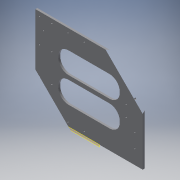
# Autodesk Inventor part: BasePlate
Saved by Autodesk Inventor 2016 (Build 200138000, 138)
## iProperties
Created: 2016-04-23
Part Number: BasePlate
Material: Generic
Document SubType Name: Modeling
Designer: Scott
Density: 1 g/cm^3
Appearance: Default
Author: Scott
Autodesk Inventor part; units mm, degrees
ref_plane "YZ Plane" through (0, 0, 0) normal (1, 0, 0) x (0, 1, 0)
ref_plane "XZ Plane" through (0, 0, 0) normal (0, 1, 0) x (-1, 0, 0)
ref_plane "XY Plane" through (0, 0, 0) normal (0, 0, 1) x (1, 0, 0)
ref_plane "Work Plane1" through (0, 0, 0) normal (0, 0, 1) x (1, 0, 0)
sketch "Sketch1" plane through (0, 0, 0) normal (0, 0, 1) x (1, 0, 0)
  line L0 (0, 273.904) -> (158.3386, 273.904)
  line L1 (133.9788, 273.904) -> (133.9788, 6.096)
  line L2 (-34.2962, 6.096) -> (302.2538, 6.096)
  line L3 (302.2538, 6.096) -> (302.2538, 273.904)
  line L4 (302.2538, 273.904) -> (-34.2962, 273.904)
  line L5 (-34.2962, 273.904) -> (-34.2962, 6.096)
  line L6 (-34.2962, 6.096) -> (302.2538, 273.904) construction
  line L7 (302.2538, 6.096) -> (-34.2962, 273.904) construction
  point P0 (0, 0)
  point P1 (0, 6.096)
  point P2 (133.9788, 140)
  dimension "d0" = 336.55
  constraints: 16 end point, 3 midpoint, 2 horizontal, 2 parallel, 1 perpendicular, 1 point on line, 1 vertical, 2 other
  measures "d0" distance of L4.end L3.end
extrude "Extrusion1" add sketch "Sketch1" against normal blind 6.096
sketch "Sketch2" plane through (0, 0, -6.096) normal (0, 0, -1) x (-1, 0, 0)
  line L0 (-302.2538, 6.096) -> (34.2962, 6.096) projected
  line L1 (34.2962, 6.096) -> (34.2962, 273.904) projected
  line L2 (34.2962, 273.904) -> (-302.2538, 273.904) projected
  line L3 (-302.2538, 273.904) -> (-302.2538, 6.096) projected
  line L4 (34.2962, 6.096) -> (-16.5038, 6.096)
  line L5 (-302.2538, 6.096) -> (34.2962, 6.096) projected
  line L6 (-16.5038, 6.096) -> (-67.3038, 6.096)
  line L7 (-67.3038, 6.096) -> (-118.1038, 6.096)
  line L8 (-16.5038, 6.096) -> (-16.5038, 18.796)
  circle A0 centre (-16.5038, 18.796) radius 2.2225
  circle A1 centre (-118.1038, 18.796) radius 2.2225
  circle A2 centre (-67.3038, 18.796) radius 2.2225
  line L9 (-16.5038, 18.796) -> (21.5962, 18.796)
  circle A3 centre (21.5962, 18.796) radius 2.2225
  line L10 (34.2962, 6.096) -> (34.2962, 273.904) projected
  line L11 (34.2962, 140) -> (8.8962, 140)
  line L12 (34.2962, 273.904) -> (-16.5038, 273.904)
  line L13 (-16.5038, 273.904) -> (-67.3038, 273.904)
  line L14 (-67.3038, 273.904) -> (-118.1038, 273.904)
  line L15 (-16.5038, 273.904) -> (-16.5038, 261.204)
  circle A4 centre (-16.5038, 261.204) radius 2.2225
  circle A5 centre (-118.1038, 261.204) radius 2.2225
  circle A6 centre (-67.3038, 261.204) radius 2.2225
  line L16 (-16.5038, 261.204) -> (21.5962, 261.204)
  circle A7 centre (21.5962, 261.204) radius 2.2225
  point P0 (0, 0)
  point P1 (0, 280)
  dimension "d3" = 50.8
  dimension "d4" = 50.8
  dimension "d5" = 50.8
  dimension "d6" = 12.7
  dimension "d7" = 4.445
  dimension "d8" = 4.445
  dimension "d9" = 4.445
  dimension "d10" = 38.1
  dimension "d11" = 4.445
  constraints: 22 end point, 10 symmetric about line, 8 centre point, 4 coincident, 3 point on line, 2 horizontal, 1 midpoint, 1 vertical, 4 other
  measures "d3" distance of L0.end L4.end
  measures "d4" distance of L4.end L6.end
  measures "d5" distance of L6.end L7.end
  measures "d6" distance of L4.end L8.end
  measures "d7" diameter of A0
  measures "d8" diameter of A1
  measures "d9" diameter of A2
  measures "d10" distance of L9.start L9.end
  measures "d11" diameter of A3
extrude "Extrusion2" cut sketch "Sketch2" against normal blind 10.8585 contours A0 L9 L8 | L8 L9 A0 | A1 | A2 | A3 | A4 L16 L15 | L15 L16 A4 | A5 | A6 | A7
sketch "Sketch3" plane through (0, 0, -6.096) normal (0, 0, -1) x (-1, 0, 0)
  circle A0 centre (-67.3038, 261.204) radius 2.2225 projected
  circle A1 centre (21.5962, 261.204) radius 2.2225 projected
  circle A2 centre (-67.3038, 18.796) radius 2.2225 projected
  circle A3 centre (-16.5038, 18.796) radius 2.2225 projected
  circle A4 centre (-118.1038, 18.796) radius 2.2225 projected
  circle A5 centre (21.5962, 18.796) radius 2.2225 projected
  circle A6 centre (-16.5038, 261.204) radius 2.2225 projected
  circle A7 centre (-118.1038, 261.204) radius 2.2225 projected
  line L0 (-302.2538, 6.096) -> (34.2962, 6.096) projected
  line L1 (34.2962, 6.096) -> (34.2962, 273.904) projected
  line L2 (34.2962, 273.904) -> (-302.2538, 273.904) projected
  line L3 (-302.2538, 273.904) -> (-302.2538, 6.096) projected
  circle A8 centre (8.8962, 228.9) radius 2.2225
  circle A9 centre (21.5962, 184.45) radius 2.2225
  circle A10 centre (-16.5038, 184.45) radius 2.2225
  circle A11 centre (-16.5038, 95.55) radius 2.2225
  circle A12 centre (8.8962, 51.1) radius 2.2225
  circle A13 centre (21.5962, 95.55) radius 2.2225
  point P0 (0, 0)
  dimension "d20" = 4.445
  dimension "d21" = 4.445
  dimension "d22" = 4.445
  dimension "d23" = 4.445
  dimension "d24" = 4.445
  dimension "d25" = 4.445
  constraints: 6 centre point
  measures "d20" diameter of A8
  measures "d21" diameter of A9
  measures "d22" diameter of A10
  measures "d23" diameter of A11
  measures "d24" diameter of A12
  measures "d25" diameter of A13
extrude "Extrusion3" cut sketch "Sketch3" against normal blind 10.8585 contours A8 | A9 | A10 | A11 | A12 | A13
sketch "Sketch4" plane through (0, 0, -6.096) normal (0, 0, -1) x (-1, 0, 0)
  circle A0 centre (8.8962, 51.1) radius 2.2225 projected
  circle A1 centre (-16.5038, 184.45) radius 2.2225 projected
  circle A2 centre (8.8962, 228.9) radius 2.2225 projected
  circle A3 centre (21.5962, 184.45) radius 2.2225 projected
  circle A4 centre (-16.5038, 95.55) radius 2.2225 projected
  circle A5 centre (21.5962, 95.55) radius 2.2225 projected
  circle A6 centre (-67.3038, 261.204) radius 2.2225 projected
  circle A7 centre (21.5962, 261.204) radius 2.2225 projected
  circle A8 centre (-67.3038, 18.796) radius 2.2225 projected
  circle A9 centre (-16.5038, 18.796) radius 2.2225 projected
  circle A10 centre (-118.1038, 18.796) radius 2.2225 projected
  circle A11 centre (21.5962, 18.796) radius 2.2225 projected
  circle A12 centre (-16.5038, 261.204) radius 2.2225 projected
  circle A13 centre (-118.1038, 261.204) radius 2.2225 projected
  line L0 (-302.2538, 6.096) -> (34.2962, 6.096) projected
  line L1 (34.2962, 6.096) -> (34.2962, 273.904) projected
  line L2 (34.2962, 273.904) -> (-302.2538, 273.904) projected
  line L3 (-302.2538, 273.904) -> (-302.2538, 6.096) projected
  line L4 (-302.2538, 6.096) -> (-302.2538, 273.904) projected
  line L5 (-302.2538, 228.9) -> (-276.8538, 228.9) construction
  line L6 (-302.2538, 140) -> (-241.6696, 140)
  circle A14 centre (-276.8538, 228.9) radius 2.2225
  circle A15 centre (-276.8538, 184.45) radius 2.2225
  circle A16 centre (-276.8538, 95.55) radius 2.2225
  circle A17 centre (-276.8538, 51.1) radius 2.2225
  line L7 (-276.8538, 184.45) -> (-238.7538, 184.45) construction
  circle A18 centre (-249.9131, 157.5092) radius 2.2225
  circle A19 centre (-249.9131, 122.4908) radius 2.2225
  point P0 (0, 0)
  dimension "d31" = 4.445
  dimension "d32" = 4.445
  dimension "d33" = 4.445
  dimension "d37" = 4.445
  dimension "d38" = 4.445
  constraints: 6 centre point, 6 end point, 3 horizontal, 1 coincident, 1 midpoint, 1 point on line
  measures "d31" diameter of A15
  measures "d32" diameter of A16
  measures "d33" diameter of A17
  measures "d37" diameter of A18
  measures "d38" diameter of A19
extrude "Extrusion4" cut sketch "Sketch4" against normal blind 10.8585 contours A14 | A15 | A16 | A17 | A18 | A19
sketch "Sketch5" plane through (0, 0, 0) normal (0, 0, 1) x (1, 0, 0)
  line L0 (253.9788, 60) -> (13.9788, 60) projected
  line L1 (13.9788, 60) -> (13.9788, 220) projected
  line L2 (13.9788, 220) -> (253.9788, 220) projected
  line L3 (253.9788, 220) -> (253.9788, 60) projected
  line L4 (37.6584, 66.1088) -> (230.2993, 66.1088)
  line L5 (230.2993, 66.1088) -> (230.2993, 213.8912)
  line L6 (230.2993, 213.8912) -> (37.6584, 213.8912)
  line L7 (37.6584, 213.8912) -> (37.6584, 66.1088)
  line L8 (37.6584, 66.1088) -> (230.2993, 213.8912) construction
  line L9 (230.2993, 66.1088) -> (37.6584, 213.8912) construction
  point P0 (0, 0)
  point P1 (133.9788, 140)
  constraints: 12 end point, 2 midpoint, 2 parallel, 1 horizontal, 1 perpendicular
extrude "Extrusion5" cut sketch "Sketch5" against normal blind 10.8585 contours L7 L6 L5 L4
sketch "Sketch6" plane through (0, 0, 0) normal (0, 0, 1) x (1, 0, 0)
  line L0 (28.0721, 134.0106) -> (240.3993, 134.0106)
  line L1 (240.3993, 134.0106) -> (240.3993, 146.7106)
  line L2 (240.3993, 146.7106) -> (28.0721, 146.7106)
  line L3 (28.0721, 146.7106) -> (28.0721, 134.0106)
  line L4 (28.0721, 134.0106) -> (240.3993, 146.7106) construction
  line L5 (240.3993, 134.0106) -> (28.0721, 146.7106) construction
  point P0 (0, 0)
  point P1 (134.2357, 140.3606)
  dimension "d43" = 12.7
  constraints: 12 end point, 2 midpoint, 2 parallel, 1 horizontal, 1 perpendicular
  measures "d43" distance of L1.end L0.end
extrude "Extrusion6" add sketch "Sketch6" against normal up to surface (6.096 mm away)
fillet "Fillet1" radius 31.75 8 edges at (230.2993, 66.1088, -3.048) (230.2993, 134.0106, -3.048) (230.2993, 146.7106, -3.048) (230.2993, 213.8912, -3.048) (37.6584, 66.1088, -3.048) (37.6584, 134.0106, -3.048) (37.6584, 146.7106, -3.048) (37.6584, 213.8912, -3.048)
body "Solid1"
